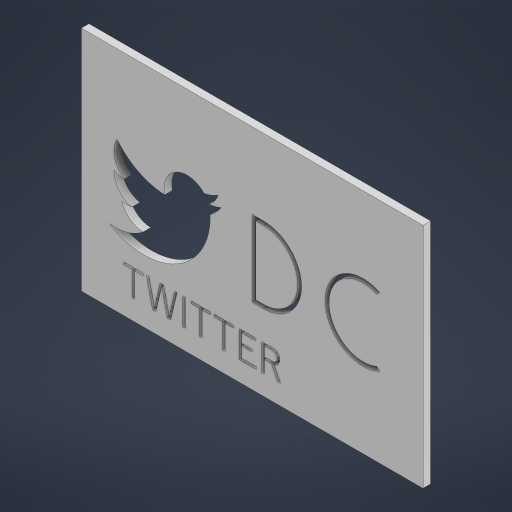
# Autodesk Inventor part: Workspacev3
Saved by Autodesk Inventor 2023.4 (Build 274418000, 418)
## iProperties
Created: 2024-02-24
Part Number: Workspacev3
Material: Generic
Document SubType Name: Modeling
Designer: ASUS
Density: 1 g/cm^3
Appearance: Default
Author: ASUS
Autodesk Inventor part; units mm, degrees
ref_plane "YZ Plane" through (0, 0, 0) normal (1, 0, 0) x (0, 1, 0)
ref_plane "XZ Plane" through (0, 0, 0) normal (0, 1, 0) x (-1, 0, 0)
ref_plane "XY Plane" through (0, 0, 0) normal (0, 0, 1) x (1, 0, 0)
sketch "Sketch3" plane through (0, 0, 0) normal (0, 0, 1) x (1, 0, 0)
  line L0 (225, -150) -> (-225, -150)
  line L1 (-225, -150) -> (-225, 150)
  line L2 (-225, 150) -> (225, 150)
  line L3 (225, 150) -> (225, -150)
  line L4 (225, -150) -> (-225, 150) construction
  line L5 (-225, -150) -> (225, 150) construction
  point P0 (0, 0)
  dimension "d28" = 450
  dimension "d29" = 300
  constraints: 12 end point, 2 midpoint, 2 parallel, 1 horizontal, 1 perpendicular
  measures "d28" distance of L1.end L2.end
  measures "d29" distance of L0.end L1.end
extrude "Extrusion3" add sketch "Sketch3" against normal blind 10
sketch "Sketch4" plane through (0, 0, 0) normal (0, 0, 1) x (1, 0, 0)
  line L0 (-188.5773, 52.7966) -> (-39.7688, 52.7966) construction
  line L1 (-39.7688, 52.7966) -> (-39.7688, -69.5636) construction
  line L2 (-39.7688, -69.5636) -> (-188.5773, -69.5636) construction
  line L3 (-188.5773, -69.5636) -> (-188.5773, 52.7966) construction
  arc A0 (-63.474, 42.3636) -> (-115.2717, 14.7448) centre (-85.6644, 21.5993) ccw
  arc A1 (-63.474, 42.3636) -> (-44.7993, 49.5387) centre (-72.9613, 94.9469) ccw
  arc A2 (-57.5211, 33.0678) -> (-44.7993, 49.5387) centre (-73.5639, 58.6073) ccw
  arc A3 (-57.5211, 33.0678) -> (-40.4668, 37.5486) centre (-61.5692, 83.1704) ccw
  arc A4 (-55.279, 22.1457) -> (-40.4668, 37.5486) centre (-91.7711, 72.0616) ccw
  arc A5 (-187.84, -54.5358) -> (-55.279, 22.1457) centre (-142.1639, 19.4243) ccw
  arc A6 (-187.84, -54.5358) -> (-143.6311, -41.8595) centre (-180.716, 4.0471) ccw
  arc A7 (-171.5212, -21.0902) -> (-143.6311, -41.8595) centre (-142.8553, -11.7068) ccw
  arc A8 (-171.5212, -21.0902) -> (-157.9673, -20.3144) centre (-166.5282, 10.4646) ccw
  arc A9 (-181.9106, 9.4083) -> (-157.9673, -20.3144) centre (-152.8099, 8.3454) ccw
  arc A10 (-181.9106, 9.4083) -> (-168.3407, 6.1387) centre (-169.5368, 30.9698) ccw
  arc A11 (-177.8021, 46.6432) -> (-168.3407, 6.1387) centre (-151.8985, 31.3367) ccw
  arc A12 (-177.8021, 46.6432) -> (-115.2717, 14.7448) centre (-111.5306, 99.3167) ccw
  line L4 (0, 50) -> (0, -50)
  line L5 (0, 50) -> (15, 50)
  line L6 (0, -50) -> (15, -50)
  arc A13 (15, -50) -> (15, 50) centre (15, 0) ccw
  line L7 (15, 45) -> (5, 45)
  line L8 (5, 45) -> (5, -45)
  line L9 (5, -45) -> (15, -45)
  arc A14 (15, -45) -> (15, 45) centre (15, 0) ccw
  arc A15 (174.4806, 41.2317) -> (167.9918, 45) centre (146.1973, 0) ccw construction
  arc A16 (164.2235, -41.2317) -> (164.2235, 41.2317) centre (146.1973, 0) ccw construction
  line L10 (167.9918, 45) -> (167.9918, -45) construction
  line L11 (167.9918, 45) -> (164.2235, 41.2317)
  line L12 (164.2235, 41.2317) -> (184.5876, 41.2317) construction
  line L13 (164.2235, 41.2317) -> (164.2235, -41.2317) construction
  line L14 (167.9918, -45) -> (164.2235, -41.2317)
  arc A17 (164.2235, 41.2317) -> (164.2235, -41.2317) centre (146.1973, 0) ccw
  arc A18 (167.9918, -45) -> (174.4806, 41.2317) centre (146.1973, 0) ccw construction
  line L15 (164.2235, -41.2317) -> (164.2235, -55.8209) construction
  arc A19 (167.9918, 45) -> (167.9918, -45) centre (146.1973, 0) ccw
  point P0 (0, 0)
  dimension "d33" = 100
  dimension "d36" = 50
  dimension "d37" = 15
  dimension "d38" = 15
  dimension "d39" = 5
  dimension "d41" = 5
  dimension "d42" = 45
  constraints: 42 point on circle, 24 end point, 20 centre point, 3 horizontal, 3 vertical, 2 point on line, 1 perpendicular, 1 tangent, 5 other
  measures "d33" distance of L4.start L4.end
  measures "d36" distance of L4.start point (0, 0)
  measures "d37" distance of L4.start L5.end
  measures "d38" distance of L4.end L6.end
  measures "d39" radial gap between concentric circles of A13 A14
  measures "d41" radial gap between concentric circles of A15 A16
  measures "d42" angle of L11 L12
extrude "Extrusion4" cut sketch "Sketch4" against normal through all
sketch "Sketch5" plane through (0, 0, 0) normal (0, 0, 1) x (1, 0, 0)
  line L0 (-171.5307, -88.98) -> (134.1497, -88.98) construction
  line L1 (134.1497, -88.98) -> (134.1497, -130.5321) construction
  line L2 (134.1497, -130.5321) -> (-171.5307, -130.5321) construction
  line L3 (-171.5307, -130.5321) -> (-171.5307, -88.98) construction
  line L4 (-143.6212, -88.98) -> (-143.6212, -91.7257)
  line L5 (-143.6212, -91.7257) -> (-154.8755, -91.7257)
  line L6 (-154.8755, -91.7257) -> (-154.8755, -123.98)
  line L7 (-154.8755, -123.98) -> (-158.0436, -123.98)
  line L8 (-158.0436, -123.98) -> (-158.0436, -91.7257)
  line L9 (-158.0436, -91.7257) -> (-169.2678, -91.7257)
  line L10 (-169.2678, -91.7257) -> (-169.2678, -88.98)
  line L11 (-169.2678, -88.98) -> (-143.6212, -88.98)
  line L12 (-98.8453, -88.98) -> (-107.354, -123.98)
  line L13 (-107.354, -123.98) -> (-111.5178, -123.98)
  line L14 (-111.5178, -123.98) -> (-116.5867, -102.3463)
  spline S0 degree 2 poles (-116.5867, -102.3463) (-117.7031, -97.6394) (-118.8195, -91.7558) knots 0 0 0 1 1 1
  line L15 (-118.8195, -91.7558) -> (-119.3324, -91.7558)
  spline S1 degree 2 poles (-119.3324, -91.7558) (-120.2074, -96.7644) (-121.535, -102.2558) knots 0 0 0 1 1 1
  line L16 (-121.535, -102.2558) -> (-126.785, -123.98)
  line L17 (-126.785, -123.98) -> (-131.0091, -123.98)
  line L18 (-131.0091, -123.98) -> (-139.1859, -88.98)
  line L19 (-139.1859, -88.98) -> (-135.8065, -88.98)
  line L20 (-135.8065, -88.98) -> (-131.16, -110.342)
  spline S2 degree 2 poles (-131.16, -110.342) (-130.4359, -113.6912) (-129.0479, -121.0532) knots 0 0 0 1 1 1
  line L21 (-129.0479, -121.0532) -> (-128.5048, -121.0532)
  spline S3 degree 2 poles (-128.5048, -121.0532) (-126.5436, -111.2472) (-126.3626, -110.5532) knots 0 0 0 1 1 1
  line L22 (-126.3626, -110.5532) -> (-121.1729, -88.98)
  line L23 (-121.1729, -88.98) -> (-116.7979, -88.98)
  line L24 (-116.7979, -88.98) -> (-111.7591, -110.7041)
  spline S4 degree 2 poles (-111.7591, -110.7041) (-111.6384, -111.217) (-109.5867, -121.0532) knots 0 0 0 1 1 1
  line L25 (-109.5867, -121.0532) -> (-109.0738, -121.0532)
  spline S5 degree 2 poles (-109.0738, -121.0532) (-108.8928, -120.1782) (-107.9876, -115.4412) knots 0 0 0 1 1 1
  spline S6 degree 2 poles (-107.9876, -115.4412) (-107.4445, -112.6955) (-106.9617, -110.6438) knots 0 0 0 1 1 1
  line L26 (-106.9617, -110.6438) -> (-102.0738, -88.98)
  line L27 (-102.0738, -88.98) -> (-98.8453, -88.98)
  line L28 (-88.104, -88.98) -> (-88.104, -123.98)
  line L29 (-88.104, -123.98) -> (-91.2721, -123.98)
  line L30 (-91.2721, -123.98) -> (-91.2721, -88.98)
  line L31 (-91.2721, -88.98) -> (-88.104, -88.98)
  line L32 (-54.7333, -88.98) -> (-54.7333, -91.7257)
  line L33 (-54.7333, -91.7257) -> (-65.9876, -91.7257)
  line L34 (-65.9876, -91.7257) -> (-65.9876, -123.98)
  line L35 (-65.9876, -123.98) -> (-69.1557, -123.98)
  line L36 (-69.1557, -123.98) -> (-69.1557, -91.7257)
  line L37 (-69.1557, -91.7257) -> (-80.3798, -91.7257)
  line L38 (-80.3798, -91.7257) -> (-80.3798, -88.98)
  line L39 (-80.3798, -88.98) -> (-54.7333, -88.98)
  line L40 (-24.5307, -88.98) -> (-24.5307, -91.7257)
  line L41 (-24.5307, -91.7257) -> (-35.785, -91.7257)
  line L42 (-35.785, -91.7257) -> (-35.785, -123.98)
  line L43 (-35.785, -123.98) -> (-38.9531, -123.98)
  line L44 (-38.9531, -123.98) -> (-38.9531, -91.7257)
  line L45 (-38.9531, -91.7257) -> (-50.1772, -91.7257)
  line L46 (-50.1772, -91.7257) -> (-50.1772, -88.98)
  line L47 (-50.1772, -88.98) -> (-24.5307, -88.98)
  line L48 (4.7064, -88.98) -> (4.7064, -91.7257)
  line L49 (4.7064, -91.7257) -> (-13.6686, -91.7257)
  line L50 (-13.6686, -91.7257) -> (-13.6686, -103.9455)
  line L51 (-13.6686, -103.9455) -> (0.2107, -103.9455)
  line L52 (0.2107, -103.9455) -> (0.2107, -106.6912)
  line L53 (0.2107, -106.6912) -> (-13.6686, -106.6912)
  line L54 (-13.6686, -106.6912) -> (-13.6686, -121.2343)
  line L55 (-13.6686, -121.2343) -> (5.0685, -121.2343)
  line L56 (5.0685, -121.2343) -> (5.0685, -123.98)
  line L57 (5.0685, -123.98) -> (-16.8367, -123.98)
  line L58 (-16.8367, -123.98) -> (-16.8367, -88.98)
  line L59 (-16.8367, -88.98) -> (4.7064, -88.98)
  line L60 (12.8831, -88.98) -> (24.3486, -88.98)
  spline S7 degree 2 poles (24.3486, -88.98) (36.1762, -88.98) (36.1762, -97.9713) knots 0 0 0 1 1 1
  spline S8 degree 2 poles (36.1762, -97.9713) (36.1762, -101.5015) (33.9736, -103.855) knots 0 0 0 1 1 1
  spline S9 degree 2 poles (33.9736, -103.855) (32.0124, -105.9972) (28.4822, -106.7515) knots 0 0 0 1 1 1
  line L61 (28.4822, -106.7515) -> (37.0512, -123.98)
  line L62 (37.0512, -123.98) -> (33.5512, -123.98)
  line L63 (33.5512, -123.98) -> (25.4952, -107.2343)
  spline S10 degree 2 poles (25.4952, -107.2343) (24.9521, -107.2946) (23.6547, -107.2946) knots 0 0 0 1 1 1
  line L64 (23.6547, -107.2946) -> (16.021, -107.2946)
  line L65 (16.021, -107.2946) -> (16.021, -123.98)
  line L66 (16.021, -123.98) -> (12.8831, -123.98)
  line L67 (12.8831, -123.98) -> (12.8831, -88.98)
  line L68 (16.021, -91.6351) -> (16.021, -104.6998)
  line L69 (16.021, -104.6998) -> (23.8357, -104.6998)
  spline S11 degree 2 poles (23.8357, -104.6998) (32.8572, -104.6998) (32.8572, -98.0015) knots 0 0 0 1 1 1
  spline S12 degree 2 poles (32.8572, -98.0015) (32.8572, -94.592) (30.5943, -93.0532) knots 0 0 0 1 1 1
  spline S13 degree 2 poles (30.5943, -93.0532) (28.4521, -91.6351) (24.1374, -91.6351) knots 0 0 0 1 1 1
  line L70 (24.1374, -91.6351) -> (16.021, -91.6351)
  point P0 (0, 0)
  constraints: 2 other
emboss "Emboss1" sketch "Sketch5" operation cut depth 100 direction (0, 0, -1)
equation "\"d37\" = d38"
equation "\"d36\" = 0.5 * d33"
body "Solid2"
